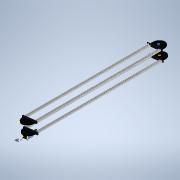
# Autodesk Inventor part: 2040ext 2200m
Saved by Autodesk Inventor 2020 (Build 240168000, 168)
## iProperties
Created: 2020-07-11
Part Number: 2040ext 2200m
Material: Aluminum 6061
Document SubType Name: Modeling
Designer: Vikki
Density: 2.7 g/cm^3
Appearance: Orange
Mass: 14268.3 g
Surface Area: 29410.2 cm^2
Volume: 5284.56 cm^3
Author: Vikki
Autodesk Inventor part; units mm, degrees
ref_plane "YZ Plane" through (0, 0, 0) normal (1, 0, 0) x (0, 1, 0)
ref_plane "XZ Plane" through (0, 0, 0) normal (0, 1, 0) x (-1, 0, 0)
ref_plane "XY Plane" through (0, 0, 0) normal (0, 0, 1) x (1, 0, 0)
sketch "Sketch1" plane through (0, 0, 0) normal (0, 0, 1) x (1, 0, 0)
  arc A0 (-9.9892, 18.3204) -> (-8.3204, 17.0108) centre (-8.5, 18.5) ccw projected
  line L0 (-8.3204, 17.0108) -> (-3.4557, 17.5974) projected
  line L1 (-3.4557, 17.5974) -> (-3.5395, 18.2923) projected
  arc A1 (-3.3648, 18.5148) -> (-3.5395, 18.2923) centre (-3.3409, 18.3163) ccw projected
  line L2 (-3.3648, 18.5148) -> (-3.067, 18.5507) projected
  line L3 (-3.067, 18.5507) -> (-3.1747, 19.4443) projected
  line L4 (-3.1747, 19.4443) -> (-5.5078, 19.163) projected
  line L5 (-5.5078, 19.163) -> (-5.7355, 21.0508) projected
  line L6 (-5.7355, 21.0508) -> (-3.6413, 23.7192) projected
  line L7 (-3.6413, 23.7192) -> (2.4177, 24.4497) projected
  line L8 (2.4177, 24.4497) -> (5.0861, 22.3556) projected
  line L9 (5.0861, 22.3556) -> (5.3138, 20.4678) projected
  line L10 (5.3138, 20.4678) -> (2.9807, 20.1865) projected
  line L11 (2.9807, 20.1865) -> (3.0884, 19.2929) projected
  line L12 (3.0884, 19.2929) -> (3.3863, 19.3289) projected
  arc A2 (3.6088, 19.1542) -> (3.3863, 19.3289) centre (3.4102, 19.1303) ccw projected
  line L13 (3.6088, 19.1542) -> (3.6926, 18.4593) projected
  line L14 (3.6926, 18.4593) -> (16.4005, 19.9915) projected
  line L15 (16.4005, 19.9915) -> (16.3167, 20.6865) projected
  arc A3 (16.4913, 20.909) -> (16.3167, 20.6865) centre (16.5153, 20.7105) ccw projected
  line L16 (16.4913, 20.909) -> (16.7892, 20.9449) projected
  line L17 (16.7892, 20.9449) -> (16.6814, 21.8385) projected
  line L18 (16.6814, 21.8385) -> (14.3483, 21.5571) projected
  line L19 (14.3483, 21.5571) -> (14.1207, 23.4449) projected
  line L20 (14.1207, 23.4449) -> (16.2149, 26.1133) projected
  line L21 (16.2149, 26.1133) -> (22.2739, 26.8439) projected
  line L22 (22.2739, 26.8439) -> (24.9423, 24.7498) projected
  line L23 (24.9423, 24.7498) -> (25.17, 22.862) projected
  line L24 (25.17, 22.862) -> (22.8369, 22.5807) projected
  line L25 (22.8369, 22.5807) -> (22.9446, 21.6871) projected
  line L26 (22.9446, 21.6871) -> (23.2424, 21.723) projected
  arc A4 (23.4649, 21.5484) -> (23.2424, 21.723) centre (23.2664, 21.5245) ccw projected
  line L27 (23.4649, 21.5484) -> (23.5487, 20.8535) projected
  line L28 (23.5487, 20.8535) -> (28.4135, 21.44) projected
  arc A5 (28.4135, 21.44) -> (29.7231, 23.1088) centre (28.2339, 22.9292) ccw projected
  line L29 (29.7231, 23.1088) -> (29.1366, 27.9736) projected
  line L30 (29.1366, 27.9736) -> (28.4416, 27.8898) projected
  arc A6 (28.2191, 28.0644) -> (28.4416, 27.8898) centre (28.4177, 28.0883) ccw projected
  line L31 (28.2191, 28.0644) -> (28.1832, 28.3622) projected
  line L32 (28.1832, 28.3622) -> (27.2897, 28.2545) projected
  line L33 (27.2897, 28.2545) -> (27.571, 25.9214) projected
  line L34 (27.571, 25.9214) -> (25.6832, 25.6938) projected
  line L35 (25.6832, 25.6938) -> (23.0148, 27.7879) projected
  line L36 (23.0148, 27.7879) -> (22.2842, 33.847) projected
  line L37 (22.2842, 33.847) -> (24.3783, 36.5154) projected
  line L38 (24.3783, 36.5154) -> (26.2661, 36.743) projected
  line L39 (26.2661, 36.743) -> (26.5475, 34.4099) projected
  line L40 (26.5475, 34.4099) -> (27.441, 34.5177) projected
  line L41 (27.441, 34.5177) -> (27.4051, 34.8155) projected
  arc A7 (27.5797, 35.038) -> (27.4051, 34.8155) centre (27.6036, 34.8394) ccw projected
  line L42 (27.5797, 35.038) -> (28.2747, 35.1218) projected
  line L43 (28.2747, 35.1218) -> (27.6881, 39.9866) projected
  arc A8 (27.6881, 39.9866) -> (26.0193, 41.2962) centre (26.1989, 39.807) ccw projected
  line L44 (26.0193, 41.2962) -> (21.1545, 40.7096) projected
  line L45 (21.1545, 40.7096) -> (21.2383, 40.0147) projected
  arc A9 (21.0637, 39.7922) -> (21.2383, 40.0147) centre (21.0398, 39.9907) ccw projected
  line L46 (21.0637, 39.7922) -> (20.7659, 39.7563) projected
  line L47 (20.7659, 39.7563) -> (20.8736, 38.8627) projected
  line L48 (20.8736, 38.8627) -> (23.2067, 39.144) projected
  line L49 (23.2067, 39.144) -> (23.4343, 37.2562) projected
  line L50 (23.4343, 37.2562) -> (21.3826, 34.6418) projected
  line L51 (21.3826, 34.6418) -> (15.2271, 33.8996) projected
  line L52 (15.2271, 33.8996) -> (12.6127, 35.9514) projected
  line L53 (12.6127, 35.9514) -> (12.3851, 37.8392) projected
  line L54 (12.3851, 37.8392) -> (14.7182, 38.1205) projected
  line L55 (14.7182, 38.1205) -> (14.6105, 39.0141) projected
  line L56 (14.6105, 39.0141) -> (14.3126, 38.9781) projected
  arc A10 (14.0901, 39.1528) -> (14.3126, 38.9781) centre (14.2887, 39.1767) ccw projected
  line L57 (14.0901, 39.1528) -> (14.0063, 39.8477) projected
  line L58 (14.0063, 39.8477) -> (1.2984, 38.3154) projected
  line L59 (1.2984, 38.3154) -> (1.3822, 37.6205) projected
  arc A11 (1.2075, 37.398) -> (1.3822, 37.6205) centre (1.1836, 37.5965) ccw projected
  line L60 (1.2075, 37.398) -> (0.9097, 37.3621) projected
  line L61 (0.9097, 37.3621) -> (1.0174, 36.4685) projected
  line L62 (1.0174, 36.4685) -> (3.3505, 36.7499) projected
  line L63 (3.3505, 36.7499) -> (3.5782, 34.8621) projected
  line L64 (3.5782, 34.8621) -> (1.5264, 32.2476) projected
  line L65 (1.5264, 32.2476) -> (-4.629, 31.5054) projected
  line L66 (-4.629, 31.5054) -> (-7.2435, 33.5572) projected
  line L67 (-7.2435, 33.5572) -> (-7.4711, 35.445) projected
  line L68 (-7.4711, 35.445) -> (-5.138, 35.7263) projected
  line L69 (-5.138, 35.7263) -> (-5.2457, 36.6199) projected
  line L70 (-5.2457, 36.6199) -> (-5.5436, 36.584) projected
  arc A12 (-5.7661, 36.7586) -> (-5.5436, 36.584) centre (-5.5675, 36.7825) ccw projected
  line L71 (-5.7661, 36.7586) -> (-5.8499, 37.4535) projected
  line L72 (-5.8499, 37.4535) -> (-10.7146, 36.867) projected
  arc A13 (-10.7146, 36.867) -> (-12.0243, 35.1982) centre (-10.5351, 35.3778) ccw projected
  line L73 (-12.0243, 35.1982) -> (-11.4377, 30.3334) projected
  line L74 (-11.4377, 30.3334) -> (-10.7427, 30.4172) projected
  arc A14 (-10.5202, 30.2426) -> (-10.7427, 30.4172) centre (-10.7188, 30.2187) ccw projected
  line L75 (-10.5202, 30.2426) -> (-10.4843, 29.9448) projected
  line L76 (-10.4843, 29.9448) -> (-9.5908, 30.0525) projected
  line L77 (-9.5908, 30.0525) -> (-9.8721, 32.3856) projected
  line L78 (-9.8721, 32.3856) -> (-7.9843, 32.6132) projected
  line L79 (-7.9843, 32.6132) -> (-5.3159, 30.5191) projected
  line L80 (-5.3159, 30.5191) -> (-4.5853, 24.46) projected
  line L81 (-4.5853, 24.46) -> (-6.6795, 21.7916) projected
  line L82 (-6.6795, 21.7916) -> (-8.5673, 21.564) projected
  line L83 (-8.5673, 21.564) -> (-8.8486, 23.8971) projected
  line L84 (-8.8486, 23.8971) -> (-9.7421, 23.7893) projected
  line L85 (-9.7421, 23.7893) -> (-9.7062, 23.4915) projected
  arc A15 (-9.8808, 23.269) -> (-9.7062, 23.4915) centre (-9.9048, 23.4676) ccw projected
  line L86 (-9.8808, 23.269) -> (-10.5758, 23.1852) projected
  line L87 (-10.5758, 23.1852) -> (-9.9892, 18.3204) projected
  line L88 (12.8698, 23.7948) -> (13.157, 21.4135) projected
  line L89 (13.157, 21.4135) -> (6.5051, 20.6114) projected
  line L90 (6.5051, 20.6114) -> (6.218, 22.9927) projected
  line L91 (6.218, 22.9927) -> (3.1586, 25.3937) projected
  line L92 (3.1586, 25.3937) -> (2.428, 31.4528) projected
  line L93 (2.428, 31.4528) -> (4.829, 34.5122) projected
  line L94 (4.829, 34.5122) -> (4.5419, 36.8935) projected
  line L95 (4.5419, 36.8935) -> (11.1937, 37.6956) projected
  line L96 (11.1937, 37.6956) -> (11.4809, 35.3143) projected
  line L97 (11.4809, 35.3143) -> (14.5403, 32.9133) projected
  line L98 (14.5403, 32.9133) -> (15.2709, 26.8542) projected
  line L99 (15.2709, 26.8542) -> (12.8698, 23.7948) projected
  circle A16 centre (-1.0787, 27.9564) radius 2.5 projected
  circle A17 centre (18.7775, 30.3506) radius 2.5 projected
  point P0 (0, 0)
extrude "Extrusion1" add sketch "Sketch1" along normal blind 2100
sketch3d "3D Sketch1"
pattern_linear "Rectangular Pattern1" count 2 spacing 150 along (0.1197094, -0.992809, 0) of "Extrusion1"
pattern_linear "Rectangular Pattern2" count 2 spacing 180 along (0.992809, 0.1197094, 0) of "Extrusion1", "Rectangular Pattern1"
sketch "Sketch2" plane through (0, 0, 0) normal (0, 0, -1) x (-1, 0, 0)
  line L0 (23.329, 45.4184) -> (0.5842, -143.2153)
  line L1 (0.5842, -143.2153) -> (-237.6899, -114.4851)
  line L2 (-237.6899, -114.4851) -> (-214.9451, 74.1486)
  line L3 (-214.9451, 74.1486) -> (23.329, 45.4184)
  line L4 (-21.649, -130.4621) -> (-34.3569, -128.9298) projected
  line L5 (-5.9321, -113.7232) -> (-6.5187, -118.5879) projected
  line L6 (-200.3546, -108.9144) -> (-213.0625, -107.3821) projected
  line L7 (-206.9803, 56.6695) -> (-206.3937, 61.5343) projected
  line L8 (-192.7119, 61.3954) -> (-180.004, 59.8631) projected
  line L9 (-219.135, 39.4003) -> (19.1392, 10.6701)
  line L10 (-182.3982, 40.007) -> (-195.1061, 41.5392) projected
  line L11 (4.7741, -108.467) -> (-233.5001, -79.7367)
  line L12 (-31.9627, -109.0736) -> (-19.2548, -110.6059) projected
  point P0 (0, 0)
  dimension "d8" = 10
  dimension "d9" = 10
  dimension "d10" = 10
  dimension "d11" = 10
  dimension "d12" = 5
  dimension "d13" = 5
  constraints: 12 end point, 4 parallel, 4 point on line, 2 perpendicular
  measures "d8" distance between parallel lines of L0 L5
  measures "d9" distance between parallel lines of L1 L6
  measures "d10" distance between parallel lines of L2 L7
  measures "d11" distance between parallel lines of L3 L8
  measures "d12" distance between parallel lines of L9 L10
  measures "d13" distance between parallel lines of L11 L12
extrude "Extrusion2" add sketch "Sketch2" along normal blind 15 contours L0 L9 L2 L3 | L0 L1 L2 L11
ref_plane "Work Plane2" through (116.1587, -108.994, 1035) normal (0.1197094, -0.992809, 0) x (-0.992809, -0.1197094, 0)
sketch "Sketch3" plane through (116.1587, -108.994, 1035) normal (0.1197094, -0.992809, 0) x (-0.992809, -0.1197094, 0)
  arc A0 (100, 1100) -> (-100, 1100) centre (0, 1100) ccw projected
  circle A1 centre (0, 1100) radius 20 projected
  arc A2 (100, 1100) -> (-100, 1100) centre (0, 1100) ccw projected
  line L0 (100, 1100) -> (100, -1100) projected
  line L1 (-100, -1100) -> (-100, 1100) projected
  line L2 (-120, 1050) -> (120, 1050) projected
  point P0 (102.2757, 1035)
  point P1 (-100, 1050)
  point P2 (100, 1050)
extrude "Extrusion3" add sketch "Sketch3" against normal mid plane 20
ref_plane "Work Plane3" through (116.1587, -108.994, 1035) normal (0.1197094, -0.992809, 0) x (-0.992809, -0.1197094, 0)
sketch "Sketch4" plane through (116.1587, -108.994, 1035) normal (0.1197094, -0.992809, 0) x (-0.992809, -0.1197094, 0)
  circle A0 centre (0, 1100) radius 20 projected
  point P0 (102.2757, 1035)
extrude "Extrusion4" add sketch "Sketch4" along normal blind 20
pattern_linear "Rectangular Pattern3" count 2 spacing 150 along (-0.1197094, 0.992809, 0) of "Extrusion3"
sketch "Sketch5" plane through (198.6802, 41.9702, -65) normal (0.1197094, -0.992809, 0) x (0.992809, 0.1197094, 0)
  line L0 (0, 50) -> (0, 0) projected
  arc A0 (-200, 0) -> (0, 0) centre (-100, 0) ccw projected
  line L1 (-200, 0) -> (-200, 50) projected
  line L2 (0, 50) -> (-200, 50) projected
  circle A1 centre (-100, 0) radius 20 projected
  point P0 (-202.2757, 65)
extrude "Extrusion5" add sketch "Sketch5" against normal blind 30 contours A1
sketch "Sketch6" plane through (21.649, -130.4621, 2100) normal (0, 0, 1) x (0.992809, 0.1197094, 0)
  line L0 (-23.6, -10) -> (-23.6, 25) projected
  line L1 (216.4, -10) -> (-23.6, -10) projected
  line L2 (-7.2, 0) -> (-7.2, 0.7) projected
  line L3 (-12.1, 0) -> (-7.2, 0) projected
  arc A0 (-13.6, 1.5) -> (-12.1, 0) centre (-12.1, 1.5) ccw projected
  line L4 (-13.6, 6.4) -> (-13.6, 1.5) projected
  line L5 (-12.9, 6.4) -> (-13.6, 6.4) projected
  arc A1 (-12.9, 6.4) -> (-12.7, 6.6) centre (-12.9, 6.6) ccw projected
  line L6 (-12.7, 6.9) -> (-12.7, 6.6) projected
  line L7 (-11.8, 6.9) -> (-12.7, 6.9) projected
  line L8 (-11.8, 4.55) -> (-11.8, 6.9) projected
  line L9 (-9.8985, 4.55) -> (-11.8, 4.55) projected
  line L10 (-7.5, 6.9485) -> (-9.8985, 4.55) projected
  line L11 (-7.5, 13.0515) -> (-7.5, 6.9485) projected
  line L12 (-9.8985, 15.45) -> (-7.5, 13.0515) projected
  line L13 (-11.8, 15.45) -> (-9.8985, 15.45) projected
  line L14 (-11.8, 13.1) -> (-11.8, 15.45) projected
  line L15 (-12.7, 13.1) -> (-11.8, 13.1) projected
  line L16 (-12.7, 13.4) -> (-12.7, 13.1) projected
  arc A2 (-12.7, 13.4) -> (-12.9, 13.6) centre (-12.9, 13.4) ccw projected
  line L17 (-13.6, 13.6) -> (-12.9, 13.6) projected
  line L18 (-13.6, 18.5) -> (-13.6, 13.6) projected
  arc A3 (-12.1, 20) -> (-13.6, 18.5) centre (-12.1, 18.5) ccw projected
  line L19 (-7.2, 20) -> (-12.1, 20) projected
  line L20 (-7.2, 19.3) -> (-7.2, 20) projected
  arc A4 (-7.2, 19.3) -> (-7, 19.1) centre (-7, 19.3) ccw projected
  line L21 (-6.7, 19.1) -> (-7, 19.1) projected
  line L22 (-6.7, 18.2) -> (-6.7, 19.1) projected
  line L23 (-9.05, 18.2) -> (-6.7, 18.2) projected
  line L24 (-9.05, 16.2985) -> (-9.05, 18.2) projected
  line L25 (-6.7, 13.9485) -> (-9.05, 16.2985) projected
  line L26 (-0.5, 13.9485) -> (-6.7, 13.9485) projected
  line L27 (1.85, 16.2985) -> (-0.5, 13.9485) projected
  line L28 (1.85, 18.2) -> (1.85, 16.2985) projected
  line L29 (-0.5, 18.2) -> (1.85, 18.2) projected
  line L30 (-0.5, 19.1) -> (-0.5, 18.2) projected
  line L31 (-0.2, 19.1) -> (-0.5, 19.1) projected
  arc A5 (-0.2, 19.1) -> (0, 19.3) centre (-0.2, 19.3) ccw projected
  line L32 (0, 20) -> (0, 19.3) projected
  line L33 (12.8, 20) -> (0, 20) projected
  line L34 (12.8, 19.3) -> (12.8, 20) projected
  arc A6 (12.8, 19.3) -> (13, 19.1) centre (13, 19.3) ccw projected
  line L35 (13.3, 19.1) -> (13, 19.1) projected
  line L36 (13.3, 18.2) -> (13.3, 19.1) projected
  line L37 (10.95, 18.2) -> (13.3, 18.2) projected
  line L38 (10.95, 16.2985) -> (10.95, 18.2) projected
  line L39 (13.3, 13.9485) -> (10.95, 16.2985) projected
  line L40 (19.5, 13.9485) -> (13.3, 13.9485) projected
  line L41 (21.85, 16.2985) -> (19.5, 13.9485) projected
  line L42 (21.85, 18.2) -> (21.85, 16.2985) projected
  line L43 (19.5, 18.2) -> (21.85, 18.2) projected
  line L44 (19.5, 19.1) -> (19.5, 18.2) projected
  line L45 (19.8, 19.1) -> (19.5, 19.1) projected
  arc A7 (19.8, 19.1) -> (20, 19.3) centre (19.8, 19.3) ccw projected
  line L46 (20, 20) -> (20, 19.3) projected
  line L47 (24.9, 20) -> (20, 20) projected
  arc A8 (26.4, 18.5) -> (24.9, 20) centre (24.9, 18.5) ccw projected
  line L48 (26.4, 13.6) -> (26.4, 18.5) projected
  line L49 (25.7, 13.6) -> (26.4, 13.6) projected
  arc A9 (25.7, 13.6) -> (25.5, 13.4) centre (25.7, 13.4) ccw projected
  line L50 (25.5, 13.1) -> (25.5, 13.4) projected
  line L51 (24.6, 13.1) -> (25.5, 13.1) projected
  line L52 (24.6, 15.45) -> (24.6, 13.1) projected
  line L53 (22.6985, 15.45) -> (24.6, 15.45) projected
  line L54 (20.3, 13.0515) -> (22.6985, 15.45) projected
  line L55 (20.3, 6.9485) -> (20.3, 13.0515) projected
  line L56 (22.6985, 4.55) -> (20.3, 6.9485) projected
  line L57 (24.6, 4.55) -> (22.6985, 4.55) projected
  line L58 (24.6, 6.9) -> (24.6, 4.55) projected
  line L59 (25.5, 6.9) -> (24.6, 6.9) projected
  line L60 (25.5, 6.6) -> (25.5, 6.9) projected
  arc A10 (25.5, 6.6) -> (25.7, 6.4) centre (25.7, 6.6) ccw projected
  line L61 (26.4, 6.4) -> (25.7, 6.4) projected
  line L62 (26.4, 1.5) -> (26.4, 6.4) projected
  arc A11 (24.9, 0) -> (26.4, 1.5) centre (24.9, 1.5) ccw projected
  line L63 (20, 0) -> (24.9, 0) projected
  line L64 (20, 0.7) -> (20, 0) projected
  arc A12 (20, 0.7) -> (19.8, 0.9) centre (19.8, 0.7) ccw projected
  line L65 (19.5, 0.9) -> (19.8, 0.9) projected
  line L66 (19.5, 1.8) -> (19.5, 0.9) projected
  line L67 (21.85, 1.8) -> (19.5, 1.8) projected
  line L68 (21.85, 3.7015) -> (21.85, 1.8) projected
  line L69 (19.4515, 6.1) -> (21.85, 3.7015) projected
  line L70 (13.3485, 6.1) -> (19.4515, 6.1) projected
  line L71 (10.95, 3.7015) -> (13.3485, 6.1) projected
  line L72 (10.95, 1.8) -> (10.95, 3.7015) projected
  line L73 (13.3, 1.8) -> (10.95, 1.8) projected
  line L74 (13.3, 0.9) -> (13.3, 1.8) projected
  line L75 (13, 0.9) -> (13.3, 0.9) projected
  arc A13 (13, 0.9) -> (12.8, 0.7) centre (13, 0.7) ccw projected
  line L76 (12.8, 0) -> (12.8, 0.7) projected
  line L77 (0, 0) -> (12.8, 0) projected
  line L78 (0, 0.7) -> (0, 0) projected
  arc A14 (0, 0.7) -> (-0.2, 0.9) centre (-0.2, 0.7) ccw projected
  line L79 (-0.5, 0.9) -> (-0.2, 0.9) projected
  line L80 (-0.5, 1.8) -> (-0.5, 0.9) projected
  line L81 (1.85, 1.8) -> (-0.5, 1.8) projected
  line L82 (1.85, 3.7015) -> (1.85, 1.8) projected
  line L83 (-0.5485, 6.1) -> (1.85, 3.7015) projected
  line L84 (-6.6515, 6.1) -> (-0.5485, 6.1) projected
  line L85 (-9.05, 3.7015) -> (-6.6515, 6.1) projected
  line L86 (-9.05, 1.8) -> (-9.05, 3.7015) projected
  line L87 (-6.7, 1.8) -> (-9.05, 1.8) projected
  line L88 (-6.7, 0.9) -> (-6.7, 1.8) projected
  line L89 (-7, 0.9) -> (-6.7, 0.9) projected
  arc A15 (-7, 0.9) -> (-7.2, 0.7) centre (-7, 0.7) ccw projected
  line L90 (172.8, 0) -> (172.8, 0.7) projected
  line L91 (167.9, 0) -> (172.8, 0) projected
  arc A16 (166.4, 1.5) -> (167.9, 0) centre (167.9, 1.5) ccw projected
  line L92 (166.4, 6.4) -> (166.4, 1.5) projected
  line L93 (167.1, 6.4) -> (166.4, 6.4) projected
  arc A17 (167.1, 6.4) -> (167.3, 6.6) centre (167.1, 6.6) ccw projected
  line L94 (167.3, 6.9) -> (167.3, 6.6) projected
  line L95 (168.2, 6.9) -> (167.3, 6.9) projected
  line L96 (168.2, 4.55) -> (168.2, 6.9) projected
  line L97 (170.1015, 4.55) -> (168.2, 4.55) projected
  line L98 (172.5, 6.9485) -> (170.1015, 4.55) projected
  line L99 (172.5, 13.0515) -> (172.5, 6.9485) projected
  line L100 (170.1015, 15.45) -> (172.5, 13.0515) projected
  line L101 (168.2, 15.45) -> (170.1015, 15.45) projected
  line L102 (168.2, 13.1) -> (168.2, 15.45) projected
  line L103 (167.3, 13.1) -> (168.2, 13.1) projected
  line L104 (167.3, 13.4) -> (167.3, 13.1) projected
  arc A18 (167.3, 13.4) -> (167.1, 13.6) centre (167.1, 13.4) ccw projected
  line L105 (166.4, 13.6) -> (167.1, 13.6) projected
  line L106 (166.4, 18.5) -> (166.4, 13.6) projected
  arc A19 (167.9, 20) -> (166.4, 18.5) centre (167.9, 18.5) ccw projected
  line L107 (172.8, 20) -> (167.9, 20) projected
  line L108 (172.8, 19.3) -> (172.8, 20) projected
  arc A20 (172.8, 19.3) -> (173, 19.1) centre (173, 19.3) ccw projected
  line L109 (173.3, 19.1) -> (173, 19.1) projected
  line L110 (173.3, 18.2) -> (173.3, 19.1) projected
  line L111 (170.95, 18.2) -> (173.3, 18.2) projected
  line L112 (170.95, 16.2985) -> (170.95, 18.2) projected
  line L113 (173.3, 13.9485) -> (170.95, 16.2985) projected
  line L114 (179.5, 13.9485) -> (173.3, 13.9485) projected
  line L115 (181.85, 16.2985) -> (179.5, 13.9485) projected
  line L116 (181.85, 18.2) -> (181.85, 16.2985) projected
  line L117 (179.5, 18.2) -> (181.85, 18.2) projected
  line L118 (179.5, 19.1) -> (179.5, 18.2) projected
  line L119 (179.8, 19.1) -> (179.5, 19.1) projected
  arc A21 (179.8, 19.1) -> (180, 19.3) centre (179.8, 19.3) ccw projected
  line L120 (180, 20) -> (180, 19.3) projected
  line L121 (192.8, 20) -> (180, 20) projected
  line L122 (192.8, 19.3) -> (192.8, 20) projected
  arc A22 (192.8, 19.3) -> (193, 19.1) centre (193, 19.3) ccw projected
  line L123 (193.3, 19.1) -> (193, 19.1) projected
  line L124 (193.3, 18.2) -> (193.3, 19.1) projected
  line L125 (190.95, 18.2) -> (193.3, 18.2) projected
  line L126 (190.95, 16.2985) -> (190.95, 18.2) projected
  line L127 (193.3, 13.9485) -> (190.95, 16.2985) projected
  line L128 (199.5, 13.9485) -> (193.3, 13.9485) projected
  line L129 (201.85, 16.2985) -> (199.5, 13.9485) projected
  line L130 (201.85, 18.2) -> (201.85, 16.2985) projected
  line L131 (199.5, 18.2) -> (201.85, 18.2) projected
  line L132 (199.5, 19.1) -> (199.5, 18.2) projected
  line L133 (199.8, 19.1) -> (199.5, 19.1) projected
  arc A23 (199.8, 19.1) -> (200, 19.3) centre (199.8, 19.3) ccw projected
  line L134 (200, 20) -> (200, 19.3) projected
  line L135 (204.9, 20) -> (200, 20) projected
  arc A24 (206.4, 18.5) -> (204.9, 20) centre (204.9, 18.5) ccw projected
  line L136 (206.4, 13.6) -> (206.4, 18.5) projected
  line L137 (205.7, 13.6) -> (206.4, 13.6) projected
  arc A25 (205.7, 13.6) -> (205.5, 13.4) centre (205.7, 13.4) ccw projected
  line L138 (205.5, 13.1) -> (205.5, 13.4) projected
  line L139 (204.6, 13.1) -> (205.5, 13.1) projected
  line L140 (204.6, 15.45) -> (204.6, 13.1) projected
  line L141 (202.6985, 15.45) -> (204.6, 15.45) projected
  line L142 (200.3, 13.0515) -> (202.6985, 15.45) projected
  line L143 (200.3, 6.9485) -> (200.3, 13.0515) projected
  line L144 (202.6985, 4.55) -> (200.3, 6.9485) projected
  line L145 (204.6, 4.55) -> (202.6985, 4.55) projected
  line L146 (204.6, 6.9) -> (204.6, 4.55) projected
  line L147 (205.5, 6.9) -> (204.6, 6.9) projected
  line L148 (205.5, 6.6) -> (205.5, 6.9) projected
  arc A26 (205.5, 6.6) -> (205.7, 6.4) centre (205.7, 6.6) ccw projected
  line L149 (206.4, 6.4) -> (205.7, 6.4) projected
  line L150 (206.4, 1.5) -> (206.4, 6.4) projected
  arc A27 (204.9, 0) -> (206.4, 1.5) centre (204.9, 1.5) ccw projected
  line L151 (200, 0) -> (204.9, 0) projected
  line L152 (200, 0.7) -> (200, 0) projected
  arc A28 (200, 0.7) -> (199.8, 0.9) centre (199.8, 0.7) ccw projected
  line L153 (199.5, 0.9) -> (199.8, 0.9) projected
  line L154 (199.5, 1.8) -> (199.5, 0.9) projected
  line L155 (201.85, 1.8) -> (199.5, 1.8) projected
  line L156 (201.85, 3.7015) -> (201.85, 1.8) projected
  line L157 (199.4515, 6.1) -> (201.85, 3.7015) projected
  line L158 (193.3485, 6.1) -> (199.4515, 6.1) projected
  line L159 (190.95, 3.7015) -> (193.3485, 6.1) projected
  line L160 (190.95, 1.8) -> (190.95, 3.7015) projected
  line L161 (193.3, 1.8) -> (190.95, 1.8) projected
  line L162 (193.3, 0.9) -> (193.3, 1.8) projected
  line L163 (193, 0.9) -> (193.3, 0.9) projected
  arc A29 (193, 0.9) -> (192.8, 0.7) centre (193, 0.7) ccw projected
  line L164 (192.8, 0) -> (192.8, 0.7) projected
  line L165 (180, 0) -> (192.8, 0) projected
  line L166 (180, 0.7) -> (180, 0) projected
  arc A30 (180, 0.7) -> (179.8, 0.9) centre (179.8, 0.7) ccw projected
  line L167 (179.5, 0.9) -> (179.8, 0.9) projected
  line L168 (179.5, 1.8) -> (179.5, 0.9) projected
  line L169 (181.85, 1.8) -> (179.5, 1.8) projected
  line L170 (181.85, 3.7015) -> (181.85, 1.8) projected
  line L171 (179.4515, 6.1) -> (181.85, 3.7015) projected
  line L172 (173.3485, 6.1) -> (179.4515, 6.1) projected
  line L173 (170.95, 3.7015) -> (173.3485, 6.1) projected
  line L174 (170.95, 1.8) -> (170.95, 3.7015) projected
  line L175 (173.3, 1.8) -> (170.95, 1.8) projected
  line L176 (173.3, 0.9) -> (173.3, 1.8) projected
  line L177 (173, 0.9) -> (173.3, 0.9) projected
  arc A31 (173, 0.9) -> (172.8, 0.7) centre (173, 0.7) ccw projected
  line L178 (-23.6, -10) -> (-23.6, 25) projected
  line L179 (216.4, -10) -> (-23.6, -10) projected
  line L180 (216.4, 25) -> (216.4, -10) projected
  line L181 (-23.6, 25) -> (216.4, 25) projected
  line L182 (172.8, 150) -> (172.8, 150.7) projected
  line L183 (167.9, 150) -> (172.8, 150) projected
  arc A32 (166.4, 151.5) -> (167.9, 150) centre (167.9, 151.5) ccw projected
  line L184 (166.4, 156.4) -> (166.4, 151.5) projected
  line L185 (167.1, 156.4) -> (166.4, 156.4) projected
  arc A33 (167.1, 156.4) -> (167.3, 156.6) centre (167.1, 156.6) ccw projected
  line L186 (167.3, 156.9) -> (167.3, 156.6) projected
  line L187 (168.2, 156.9) -> (167.3, 156.9) projected
  line L188 (168.2, 154.55) -> (168.2, 156.9) projected
  line L189 (170.1015, 154.55) -> (168.2, 154.55) projected
  line L190 (172.5, 156.9485) -> (170.1015, 154.55) projected
  line L191 (172.5, 163.0515) -> (172.5, 156.9485) projected
  line L192 (170.1015, 165.45) -> (172.5, 163.0515) projected
  line L193 (168.2, 165.45) -> (170.1015, 165.45) projected
  line L194 (168.2, 163.1) -> (168.2, 165.45) projected
  line L195 (167.3, 163.1) -> (168.2, 163.1) projected
  line L196 (167.3, 163.4) -> (167.3, 163.1) projected
  arc A34 (167.3, 163.4) -> (167.1, 163.6) centre (167.1, 163.4) ccw projected
  line L197 (166.4, 163.6) -> (167.1, 163.6) projected
  line L198 (166.4, 168.5) -> (166.4, 163.6) projected
  arc A35 (167.9, 170) -> (166.4, 168.5) centre (167.9, 168.5) ccw projected
  line L199 (172.8, 170) -> (167.9, 170) projected
  line L200 (172.8, 169.3) -> (172.8, 170) projected
  arc A36 (172.8, 169.3) -> (173, 169.1) centre (173, 169.3) ccw projected
  line L201 (173.3, 169.1) -> (173, 169.1) projected
  line L202 (173.3, 168.2) -> (173.3, 169.1) projected
  line L203 (170.95, 168.2) -> (173.3, 168.2) projected
  line L204 (170.95, 166.2985) -> (170.95, 168.2) projected
  line L205 (173.3, 163.9485) -> (170.95, 166.2985) projected
  line L206 (179.5, 163.9485) -> (173.3, 163.9485) projected
  line L207 (181.85, 166.2985) -> (179.5, 163.9485) projected
  line L208 (181.85, 168.2) -> (181.85, 166.2985) projected
  line L209 (179.5, 168.2) -> (181.85, 168.2) projected
  line L210 (179.5, 169.1) -> (179.5, 168.2) projected
  line L211 (179.8, 169.1) -> (179.5, 169.1) projected
  arc A37 (179.8, 169.1) -> (180, 169.3) centre (179.8, 169.3) ccw projected
  line L212 (180, 170) -> (180, 169.3) projected
  line L213 (192.8, 170) -> (180, 170) projected
  line L214 (192.8, 169.3) -> (192.8, 170) projected
  arc A38 (192.8, 169.3) -> (193, 169.1) centre (193, 169.3) ccw projected
  line L215 (193.3, 169.1) -> (193, 169.1) projected
  line L216 (193.3, 168.2) -> (193.3, 169.1) projected
  line L217 (190.95, 168.2) -> (193.3, 168.2) projected
  line L218 (190.95, 166.2985) -> (190.95, 168.2) projected
  line L219 (193.3, 163.9485) -> (190.95, 166.2985) projected
  line L220 (199.5, 163.9485) -> (193.3, 163.9485) projected
  line L221 (201.85, 166.2985) -> (199.5, 163.9485) projected
  line L222 (201.85, 168.2) -> (201.85, 166.2985) projected
  line L223 (199.5, 168.2) -> (201.85, 168.2) projected
  line L224 (199.5, 169.1) -> (199.5, 168.2) projected
  line L225 (199.8, 169.1) -> (199.5, 169.1) projected
  arc A39 (199.8, 169.1) -> (200, 169.3) centre (199.8, 169.3) ccw projected
  line L226 (200, 170) -> (200, 169.3) projected
  line L227 (204.9, 170) -> (200, 170) projected
  arc A40 (206.4, 168.5) -> (204.9, 170) centre (204.9, 168.5) ccw projected
  line L228 (206.4, 163.6) -> (206.4, 168.5) projected
  line L229 (205.7, 163.6) -> (206.4, 163.6) projected
  arc A41 (205.7, 163.6) -> (205.5, 163.4) centre (205.7, 163.4) ccw projected
  line L230 (205.5, 163.1) -> (205.5, 163.4) projected
  line L231 (204.6, 163.1) -> (205.5, 163.1) projected
  line L232 (204.6, 165.45) -> (204.6, 163.1) projected
  line L233 (202.6985, 165.45) -> (204.6, 165.45) projected
  line L234 (200.3, 163.0515) -> (202.6985, 165.45) projected
  line L235 (200.3, 156.9485) -> (200.3, 163.0515) projected
  line L236 (202.6985, 154.55) -> (200.3, 156.9485) projected
  line L237 (204.6, 154.55) -> (202.6985, 154.55) projected
  line L238 (204.6, 156.9) -> (204.6, 154.55) projected
  line L239 (205.5, 156.9) -> (204.6, 156.9) projected
  line L240 (205.5, 156.6) -> (205.5, 156.9) projected
  arc A42 (205.5, 156.6) -> (205.7, 156.4) centre (205.7, 156.6) ccw projected
  line L241 (206.4, 156.4) -> (205.7, 156.4) projected
  line L242 (206.4, 151.5) -> (206.4, 156.4) projected
  arc A43 (204.9, 150) -> (206.4, 151.5) centre (204.9, 151.5) ccw projected
  line L243 (200, 150) -> (204.9, 150) projected
  line L244 (200, 150.7) -> (200, 150) projected
  arc A44 (200, 150.7) -> (199.8, 150.9) centre (199.8, 150.7) ccw projected
  line L245 (199.5, 150.9) -> (199.8, 150.9) projected
  line L246 (199.5, 151.8) -> (199.5, 150.9) projected
  line L247 (201.85, 151.8) -> (199.5, 151.8) projected
  line L248 (201.85, 153.7015) -> (201.85, 151.8) projected
  line L249 (199.4515, 156.1) -> (201.85, 153.7015) projected
  line L250 (193.3485, 156.1) -> (199.4515, 156.1) projected
  line L251 (190.95, 153.7015) -> (193.3485, 156.1) projected
  line L252 (190.95, 151.8) -> (190.95, 153.7015) projected
  line L253 (193.3, 151.8) -> (190.95, 151.8) projected
  line L254 (193.3, 150.9) -> (193.3, 151.8) projected
  line L255 (193, 150.9) -> (193.3, 150.9) projected
  arc A45 (193, 150.9) -> (192.8, 150.7) centre (193, 150.7) ccw projected
  line L256 (192.8, 150) -> (192.8, 150.7) projected
  line L257 (180, 150) -> (192.8, 150) projected
  line L258 (180, 150.7) -> (180, 150) projected
  arc A46 (180, 150.7) -> (179.8, 150.9) centre (179.8, 150.7) ccw projected
  line L259 (179.5, 150.9) -> (179.8, 150.9) projected
  line L260 (179.5, 151.8) -> (179.5, 150.9) projected
  line L261 (181.85, 151.8) -> (179.5, 151.8) projected
  line L262 (181.85, 153.7015) -> (181.85, 151.8) projected
  line L263 (179.4515, 156.1) -> (181.85, 153.7015) projected
  line L264 (173.3485, 156.1) -> (179.4515, 156.1) projected
  line L265 (170.95, 153.7015) -> (173.3485, 156.1) projected
  line L266 (170.95, 151.8) -> (170.95, 153.7015) projected
  line L267 (173.3, 151.8) -> (170.95, 151.8) projected
  line L268 (173.3, 150.9) -> (173.3, 151.8) projected
  line L269 (173, 150.9) -> (173.3, 150.9) projected
  arc A47 (173, 150.9) -> (172.8, 150.7) centre (173, 150.7) ccw projected
  line L270 (-7.2, 150) -> (-7.2, 150.7) projected
  line L271 (-12.1, 150) -> (-7.2, 150) projected
  arc A48 (-13.6, 151.5) -> (-12.1, 150) centre (-12.1, 151.5) ccw projected
  line L272 (-13.6, 156.4) -> (-13.6, 151.5) projected
  line L273 (-12.9, 156.4) -> (-13.6, 156.4) projected
  arc A49 (-12.9, 156.4) -> (-12.7, 156.6) centre (-12.9, 156.6) ccw projected
  line L274 (-12.7, 156.9) -> (-12.7, 156.6) projected
  line L275 (-11.8, 156.9) -> (-12.7, 156.9) projected
  line L276 (-11.8, 154.55) -> (-11.8, 156.9) projected
  line L277 (-9.8985, 154.55) -> (-11.8, 154.55) projected
  line L278 (-7.5, 156.9485) -> (-9.8985, 154.55) projected
  line L279 (-7.5, 163.0515) -> (-7.5, 156.9485) projected
  line L280 (-9.8985, 165.45) -> (-7.5, 163.0515) projected
  line L281 (-11.8, 165.45) -> (-9.8985, 165.45) projected
  line L282 (-11.8, 163.1) -> (-11.8, 165.45) projected
  line L283 (-12.7, 163.1) -> (-11.8, 163.1) projected
  line L284 (-12.7, 163.4) -> (-12.7, 163.1) projected
  arc A50 (-12.7, 163.4) -> (-12.9, 163.6) centre (-12.9, 163.4) ccw projected
  line L285 (-13.6, 163.6) -> (-12.9, 163.6) projected
  line L286 (-13.6, 168.5) -> (-13.6, 163.6) projected
  arc A51 (-12.1, 170) -> (-13.6, 168.5) centre (-12.1, 168.5) ccw projected
  line L287 (-7.2, 170) -> (-12.1, 170) projected
  line L288 (-7.2, 169.3) -> (-7.2, 170) projected
  arc A52 (-7.2, 169.3) -> (-7, 169.1) centre (-7, 169.3) ccw projected
  line L289 (-6.7, 169.1) -> (-7, 169.1) projected
  line L290 (-6.7, 168.2) -> (-6.7, 169.1) projected
  line L291 (-9.05, 168.2) -> (-6.7, 168.2) projected
  line L292 (-9.05, 166.2985) -> (-9.05, 168.2) projected
  line L293 (-6.7, 163.9485) -> (-9.05, 166.2985) projected
  line L294 (-0.5, 163.9485) -> (-6.7, 163.9485) projected
  line L295 (1.85, 166.2985) -> (-0.5, 163.9485) projected
  line L296 (1.85, 168.2) -> (1.85, 166.2985) projected
  line L297 (-0.5, 168.2) -> (1.85, 168.2) projected
  line L298 (-0.5, 169.1) -> (-0.5, 168.2) projected
  line L299 (-0.2, 169.1) -> (-0.5, 169.1) projected
  arc A53 (-0.2, 169.1) -> (0, 169.3) centre (-0.2, 169.3) ccw projected
  line L300 (0, 170) -> (0, 169.3) projected
  line L301 (12.8, 170) -> (0, 170) projected
  line L302 (12.8, 169.3) -> (12.8, 170) projected
  arc A54 (12.8, 169.3) -> (13, 169.1) centre (13, 169.3) ccw projected
  line L303 (13.3, 169.1) -> (13, 169.1) projected
  line L304 (13.3, 168.2) -> (13.3, 169.1) projected
  line L305 (10.95, 168.2) -> (13.3, 168.2) projected
  line L306 (10.95, 166.2985) -> (10.95, 168.2) projected
  line L307 (13.3, 163.9485) -> (10.95, 166.2985) projected
  line L308 (19.5, 163.9485) -> (13.3, 163.9485) projected
  line L309 (21.85, 166.2985) -> (19.5, 163.9485) projected
  line L310 (21.85, 168.2) -> (21.85, 166.2985) projected
  line L311 (19.5, 168.2) -> (21.85, 168.2) projected
  line L312 (19.5, 169.1) -> (19.5, 168.2) projected
  line L313 (19.8, 169.1) -> (19.5, 169.1) projected
  arc A55 (19.8, 169.1) -> (20, 169.3) centre (19.8, 169.3) ccw projected
  line L314 (20, 170) -> (20, 169.3) projected
  line L315 (24.9, 170) -> (20, 170) projected
  arc A56 (26.4, 168.5) -> (24.9, 170) centre (24.9, 168.5) ccw projected
  line L316 (26.4, 163.6) -> (26.4, 168.5) projected
  line L317 (25.7, 163.6) -> (26.4, 163.6) projected
  arc A57 (25.7, 163.6) -> (25.5, 163.4) centre (25.7, 163.4) ccw projected
  line L318 (25.5, 163.1) -> (25.5, 163.4) projected
  line L319 (24.6, 163.1) -> (25.5, 163.1) projected
  line L320 (24.6, 165.45) -> (24.6, 163.1) projected
  line L321 (22.6985, 165.45) -> (24.6, 165.45) projected
  line L322 (20.3, 163.0515) -> (22.6985, 165.45) projected
  line L323 (20.3, 156.9485) -> (20.3, 163.0515) projected
  line L324 (22.6985, 154.55) -> (20.3, 156.9485) projected
  line L325 (24.6, 154.55) -> (22.6985, 154.55) projected
  line L326 (24.6, 156.9) -> (24.6, 154.55) projected
  line L327 (25.5, 156.9) -> (24.6, 156.9) projected
  line L328 (25.5, 156.6) -> (25.5, 156.9) projected
  arc A58 (25.5, 156.6) -> (25.7, 156.4) centre (25.7, 156.6) ccw projected
  line L329 (26.4, 156.4) -> (25.7, 156.4) projected
  line L330 (26.4, 151.5) -> (26.4, 156.4) projected
  arc A59 (24.9, 150) -> (26.4, 151.5) centre (24.9, 151.5) ccw projected
  line L331 (20, 150) -> (24.9, 150) projected
  line L332 (20, 150.7) -> (20, 150) projected
  arc A60 (20, 150.7) -> (19.8, 150.9) centre (19.8, 150.7) ccw projected
  line L333 (19.5, 150.9) -> (19.8, 150.9) projected
  line L334 (19.5, 151.8) -> (19.5, 150.9) projected
  line L335 (21.85, 151.8) -> (19.5, 151.8) projected
  line L336 (21.85, 153.7015) -> (21.85, 151.8) projected
  line L337 (19.4515, 156.1) -> (21.85, 153.7015) projected
  line L338 (13.3485, 156.1) -> (19.4515, 156.1) projected
  line L339 (10.95, 153.7015) -> (13.3485, 156.1) projected
  line L340 (10.95, 151.8) -> (10.95, 153.7015) projected
  line L341 (13.3, 151.8) -> (10.95, 151.8) projected
  line L342 (13.3, 150.9) -> (13.3, 151.8) projected
  line L343 (13, 150.9) -> (13.3, 150.9) projected
  arc A61 (13, 150.9) -> (12.8, 150.7) centre (13, 150.7) ccw projected
  line L344 (12.8, 150) -> (12.8, 150.7) projected
  line L345 (0, 150) -> (12.8, 150) projected
  line L346 (0, 150.7) -> (0, 150) projected
  arc A62 (0, 150.7) -> (-0.2, 150.9) centre (-0.2, 150.7) ccw projected
  line L347 (-0.5, 150.9) -> (-0.2, 150.9) projected
  line L348 (-0.5, 151.8) -> (-0.5, 150.9) projected
  line L349 (1.85, 151.8) -> (-0.5, 151.8) projected
  line L350 (1.85, 153.7015) -> (1.85, 151.8) projected
  line L351 (-0.5485, 156.1) -> (1.85, 153.7015) projected
  line L352 (-6.6515, 156.1) -> (-0.5485, 156.1) projected
  line L353 (-9.05, 153.7015) -> (-6.6515, 156.1) projected
  line L354 (-9.05, 151.8) -> (-9.05, 153.7015) projected
  line L355 (-6.7, 151.8) -> (-9.05, 151.8) projected
  line L356 (-6.7, 150.9) -> (-6.7, 151.8) projected
  line L357 (-7, 150.9) -> (-6.7, 150.9) projected
  arc A63 (-7, 150.9) -> (-7.2, 150.7) centre (-7, 150.7) ccw projected
  line L358 (-23.6, 180) -> (216.4, 180) projected
  line L359 (-23.6, 145) -> (-23.6, 180) projected
  line L360 (216.4, 145) -> (-23.6, 145) projected
  line L361 (216.4, 180) -> (216.4, 145) projected
  point P0 (-5.8757, 132.1155)
extrude "Extrusion6" add sketch "Sketch6" along normal blind 20 contours L0 L181 L180 L1 | L3 A0 L4 L5 A1 L6 L7 L8 L9 L10 L11 L12 L13 L14 L15 L16 A2 L17 L18 A3 L19 L20 A4 L21 L22 L23 L24 L25 L26 L27 L28 L29 L30 L31 A5 L32 L33 L34 A6 L35 L36 L37 L38 L39 L40 L41 L42 L43 L44 L45 A7 L46 L47 A8 L48 L49 A9 L50 L51 L52 L53 L54 L55 L56 L57 L58 L59 L60 A10 L61 L62 A11 L63 L64 A12 L65 L66 L67 L68 L69 L70 L71 L72 L73 L74 L75 A13 L76 L77 L78 A14 L79 L80 L81 L82 L83 L84 L85 L86 L87 L88 L89 A15 L2 | L91 A16 L92 L93 A17 L94 L95 L96 L97 L98 L99 L100 L101 L102 L103 L104 A18 L105 L106 A19 L107 L108 A20 L109 L110 L111 L112 L113 L114 L115 L116 L117 L118 L119 A21 L120 L121 L122 A22 L123 L124 L125 L126 L127 L128 L129 L130 L131 L132 L133 A23 L134 L135 A24 L136 L137 A25 L138 L139 L140 L141 L142 L143 L144 L145 L146 L147 L148 A26 L149 L150 A27 L151 L152 A28 L153 L154 L155 L156 L157 L158 L159 L160 L161 L162 L163 A29 L164 L165 L166 A30 L167 L168 L169 L170 L171 L172 L173 L174 L175 L176 L177 A31 L90 | L183 A32 L184 L185 A33 L186 L187 L188 L189 L190 L191 L192 L193 L194 L195 L196 A34 L197 L198 A35 L199 L200 A36 L201 L202 L203 L204 L205 L206 L207 L208 L209 L210 L211 A37 L212 L213 L214 A38 L215 L216 L217 L218 L219 L220 L221 L222 L223 L224 L225 A39 L226 L227 A40 L228 L229 A41 L230 L231 L232 L233 L234 L235 L236 L237 L238 L239 L240 A42 L241 L242 A43 L243 L244 A44 L245 L246 L247 L248 L249 L250 L251 L252 L253 L254 L255 A45 L256 L257 L258 A46 L259 L260 L261 L262 L263 L264 L265 L266 L267 L268 L269 A47 L182 | L271 A48 L272 L273 A49 L274 L275 L276 L277 L278 L279 L280 L281 L282 L283 L284 A50 L285 L286 A51 L287 L288 A52 L289 L290 L291 L292 L293 L294 L295 L296 L297 L298 L299 A53 L300 L301 L302 A54 L303 L304 L305 L306 L307 L308 L309 L310 L311 L312 L313 A55 L314 L315 A56 L316 L317 A57 L318 L319 L320 L321 L322 L323 L324 L325 L326 L327 L328 A58 L329 L330 A59 L331 L332 A60 L333 L334 L335 L336 L337 L338 L339 L340 L341 L342 L343 A61 L344 L345 L346 A62 L347 L348 L349 L350 L351 L352 L353 L354 L355 L356 L357 A63 L270 | L358 L361 L360 L359
ref_plane "Work Plane4" through (116.1587, -108.994, 1035) normal (0.1197094, -0.992809, 0) x (-0.992809, -0.1197094, 0)
sketch "Sketch7" plane through (116.1587, -108.994, 1035) normal (0.1197094, -0.992809, 0) x (-0.992809, -0.1197094, 0)
  circle A0 centre (0, -1100) radius 20 projected
  arc A1 (-100, -1100) -> (100, -1100) centre (0, -1100) ccw projected
  line L0 (120, -1085) -> (-120, -1085) projected
  line L1 (-100, -1100) -> (-100, 1100) projected
  line L2 (100, 1100) -> (100, -1100) projected
  line L3 (100, 1100) -> (100, -1100) projected
  point P0 (102.2757, 1035)
  point P1 (100, -1085)
  point P2 (-100, -1085)
extrude "Extrusion7" add sketch "Sketch7" along normal mid plane 20 contours A0 L0 | A0 L0 L2 A1 L1 picked at (-3.6439, -1099.8342)
pattern_linear "Rectangular Pattern4" count 2 spacing 150 along (-0.1197094, 0.992809, 0) of "Extrusion7"
sketch "Sketch8" plane through (-2.2757, 37.8845, 2135) normal (-0.1197094, 0.992809, 0) x (0.992809, 0.1197094, 0)
  point P0 (-2.2757, 2135)
sketch "Sketch9" plane through (117.3557, -118.9221, 1035) normal (0.1197094, -0.992809, 0) x (0.992809, 0.1197094, 0)
  line L0 (-36, 1085) -> (50, 1085)
  line L1 (50, 1085) -> (50, 1185)
  line L2 (50, 1185) -> (-36, 1185)
  line L3 (-36, 1185) -> (-36, 1085)
  line L4 (100, 1085) -> (100, 1100) projected
  line L5 (100, 1085) -> (-100, 1085) projected
  point P0 (-102.2757, -1035)
  dimension "d32" = 50
  dimension "d33" = 100
  dimension "d34" = 86
  dimension "d35" = 0
  constraints: 8 end point, 2 parallel, 1 horizontal, 1 perpendicular
  measures "d32" distance between parallel lines of L4 L1
  measures "d33" distance of L0.end L1.end
  measures "d34" distance of L1.end L2.end
  measures "d35" distance between parallel lines of L5 L0
extrude "Extrusion8" add sketch "Sketch9" along normal blind 50
sketch "Sketch10" plane through (81.6146, -123.2316, 2220) normal (0, 0, 1) x (0.992809, 0.1197094, 0)
  line L0 (86, 0) -> (86, -50) projected
  line L1 (0, 0) -> (0, -50) projected
  line L2 (86, -50) -> (0, 0)
  line L3 (0, 0) -> (86, 0) projected
  line L4 (0, -50) -> (86, 0)
  circle A0 centre (43, -25) radius 20
  point P0 (-66.2757, 132.1155)
  dimension "d38" = 40
  constraints: 4 end point, 1 centre point, 1 midpoint
  measures "d38" diameter of A0
sketch "Sketch11" plane through (168.1933, -122.8647, 2120) normal (0, 0, -1) x (-0.992809, -0.1197094, 0)
  circle A0 centre (43, -15) radius 20 projected
  circle A1 centre (43, -15) radius 20 projected
  point P0 (152.2757, 142.1155)
extrude "Extrusion10" add sketch "Sketch11" along normal blind 40
fillet "Fillet2" radius 2 1 edges at (147.1543, -140.5102, 2080)
sketch "Sketch12" plane through (127.2981, -142.9044, 2080) normal (0, 0, -1) x (-1, 0, 0)
  circle A0 centre (0, 0) radius 18 projected
  point P0 (127.2981, 142.9044)
extrude "Extrusion11" add sketch "Sketch12" along normal blind 60
fillet "Fillet3" radius 5 1 edges at (145.2981, -142.9044, 2020)
sketch "Sketch13" plane through (118.5528, -128.8502, -65) normal (0.1197094, -0.992809, 0) x (0.992809, 0.1197094, 0)
  line L0 (-1.8907, -3.2389) -> (17.8907, -3.2389)
  line L1 (17.8907, -3.2389) -> (17.8907, 5.2389)
  line L2 (17.8907, 5.2389) -> (-1.8907, 5.2389)
  line L3 (-1.8907, 5.2389) -> (-1.8907, -3.2389)
  line L4 (-1.8907, -3.2389) -> (17.8907, 5.2389) construction
  line L5 (17.8907, -3.2389) -> (-1.8907, 5.2389) construction
  point P0 (-102.2757, 65)
  point P1 (8, 1)
  constraints: 12 end point, 2 midpoint, 2 parallel, 1 horizontal, 1 perpendicular
extrude "Extrusion12" add sketch "Sketch13" along normal blind 5
body "Solid1"
